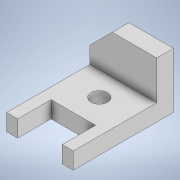
# Autodesk Inventor part: LBracket
Saved by Autodesk Inventor 2022.2 (Build 262287030, 287C)
## iProperties
Created: 2023-02-24
Part Number: LBracket
Material: Generic
Document SubType Name: Modeling
Designer: jak27277
Density: 1 g/cm^3
Appearance: Default
Author: jak27277
Autodesk Inventor part; units mm, degrees
ref_plane "YZ Plane" through (0, 0, 0) normal (1, 0, 0) x (0, 1, 0)
ref_plane "XZ Plane" through (0, 0, 0) normal (0, 1, 0) x (-1, 0, 0)
ref_plane "XY Plane" through (0, 0, 0) normal (0, 0, 1) x (1, 0, 0)
sketch "Sketch2" plane through (0, 0, 0) normal (1, 0, 0) x (0, 1, 0)
  line L0 (0, 0) -> (0, 114.3)
  line L1 (0, 114.3) -> (19.05, 114.3)
  line L2 (19.05, 114.3) -> (19.05, 19.05)
  line L3 (19.05, 19.05) -> (63.5, 19.05)
  line L4 (63.5, 19.05) -> (63.5, 0)
  line L5 (63.5, 0) -> (0, 0)
  dimension "d0" = 114.3
  dimension "d1" = 63.5
  dimension "d2" = 19.05
  constraints: 12 end point, 6 perpendicular, 1 vertical
  measures "d0" distance of L0.start L0.end
  measures "d1" distance of L4.end L0.start
  measures "d2" distance of L3.end L4.end
extrude "Extrusion1" add sketch "Sketch2" along normal mid plane 76.2
sketch "Sketch3" plane through (-38.1, 19.05, 114.3) normal (0, 1, 0) x (1, 0, 0)
  line L0 (0, 0) -> (76.2, 0) projected
  line L1 (12.7, 0) -> (63.5, 0)
  line L2 (63.5, 0) -> (63.5, 38.1)
  line L3 (63.5, 38.1) -> (12.7, 38.1)
  line L4 (12.7, 38.1) -> (12.7, 0)
  line L5 (12.7, 38.1) -> (0, 38.1) construction
  line L6 (0, 0) -> (0, 95.25) construction
  line L7 (63.5, 38.1) -> (76.2, 38.1) construction
  line L8 (76.2, 95.25) -> (76.2, 0) construction
  circle A0 centre (38.1, 67.818) radius 9.525
  point P0 (38.1, 114.3)
  point P1 (63.5, 0)
  dimension "d5" = 12.7
  dimension "d6" = 50.8
  dimension "d7" = 38.1
  dimension "d8" = 38.1
  dimension "d9" = 67.818
  dimension "d10" = 19.05
  constraints: 12 end point, 4 point on line, 2 horizontal, 2 parallel, 1 centre point, 1 perpendicular
  measures "d5" distance between parallel lines of L6 L4
  measures "d6" distance of L2.end L3.end
  measures "d7" distance of L3.end L1.start
  measures "d8" distance from line of L6 A0.centre
  measures "d9" distance from line of A0.centre L0
  measures "d10" diameter of A0
extrude "Extrusion2" cut sketch "Sketch3" against normal through all
sketch "Sketch4" plane through (-38.1, 19.05, 19.05) normal (0, 0, 1) x (1, 0, 0)
  line L0 (0, 44.45) -> (0, -19.05) projected
  line L1 (0, 19.05) -> (25.4, 44.45)
  line L2 (76.2, 44.45) -> (0, 44.45) projected
  point P0 (38.1, -19.05)
  dimension "d13" = 50.8
  dimension "d14" = 25.4
  constraints: 2 end point, 2 point on line
  measures "d13" distance of L2.start L1.end
  measures "d14" distance of L0.start L1.start
extrude "Extrusion3" cut sketch "Sketch4" against normal through all
body "Solid1"
